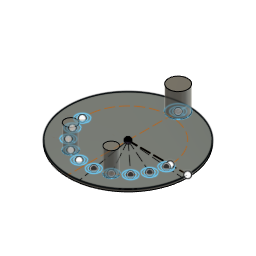
Tangible Interfaces Plate Concept (Autodesk Fusion 360 design; units mm, degrees)
Autodesk Fusion 360 part; units mm, degrees
sketch "Sketch1" plane through (0, 0, 0) normal (0, 1, 0) x (1, 0, 0)
  circle A0 centre (0, 0) radius 37.5
  line L0 (0, 37.5) -> (0, -37.5) construction
  line L1 (0, 0) -> (37.5, 0) construction
  circle A1 centre (0, 0) radius 26.5 construction
  line L2 (0, 0) -> (37.5, 0) construction
  line L3 (0, 0) -> (6.5118, -36.9303) construction
  line L4 (0, 0) -> (37.5, 0) construction
  line L5 (0, 0) -> (37.3573, -3.2683) construction
  line L6 (0, 0) -> (37.5, 0) construction
  line L7 (0, 0) -> (24.2558, -10.6728) construction
  line L8 (0, 0) -> (26.5, 0) construction
  line L9 (0, 0) -> (19.5378, -17.9031) construction
  line L10 (0, 0) -> (26.5, 0) construction
  line L11 (0, 0) -> (12.7462, -23.2333) construction
  line L12 (0, 0) -> (26.5, 0) construction
  circle A2 centre (26.3992, -2.3096) radius 2.5
  circle A3 centre (24.2558, -10.6728) radius 2.5
  circle A4 centre (19.5378, -17.9031) radius 2.5
  circle A5 centre (12.7462, -23.2333) radius 2.5
  circle A6 centre (4.6017, -26.0974) radius 2.5
  circle A7 centre (-4.6017, -26.0974) radius 2.5
  circle A8 centre (-12.7462, -23.2333) radius 2.5
  circle A9 centre (-19.5378, -17.9031) radius 2.5
  circle A10 centre (-24.2558, -10.6728) radius 2.5
  circle A11 centre (-26.3992, -2.3096) radius 2.5
  line L13 (0, 37.5) -> (0, 31.5)
  circle A12 centre (0, 31.5) radius 2.5
  circle A13 centre (-24.2558, -10.6728) radius 3.75
  circle A14 centre (24.2558, -10.6728) radius 3.75
  circle A15 centre (0, 31.5) radius 3.75
  circle A16 centre (-4.6017, -26.0974) radius 3.75
  circle A17 centre (4.6017, -26.0974) radius 3.75
  circle A18 centre (-12.7462, -23.2333) radius 3.75
  circle A19 centre (12.7462, -23.2333) radius 3.75
  circle A20 centre (-19.5378, -17.9031) radius 3.75
  circle A21 centre (-26.3992, -2.3096) radius 3.75
  circle A22 centre (26.3992, -2.3096) radius 3.75
  circle A23 centre (19.5378, -17.9031) radius 3.75
  circle A24 centre (0, 31.5) radius 6
  dimension "d1" = 75
  dimension "d5" = 80
  dimension "d6" = 5
  dimension "d9" = 23.75
  dimension "d10" = 42.5
  dimension "d11" = 61.25
  dimension "d12" = 5
  dimension "d13" = 5
  dimension "d14" = 5
  dimension "d15" = 5
  dimension "d16" = 5
  dimension "d29" = 6
  dimension "d39" = 7.5
  dimension "d40" = 7.5
  dimension "d41" = 7.5
  dimension "d44" = 7.5
  dimension "d45" = 7.5
  dimension "d46" = 7.5
  dimension "d47" = 7.5
  dimension "d52" = 7.5
  dimension "d53" = 7.5
  dimension "d58" = 7.5
  dimension "d63" = 7.5
  dimension "d66" = 12
  constraint coincident A0.centre L1.start
  constraint coincident A0 L0.start
  constraint coincident A0 L0.end
  constraint coincident A0 L1.end
  constraint perpendicular L0 L1
  constraint horizontal L2
  constraint horizontal L4
  constraint coincident A0 L3.end
  constraint horizontal L6
  constraint coincident A0 L5.end
  constraint horizontal L8
  constraint coincident A1 L7.end
  constraint horizontal L10
  constraint horizontal L12
  constraint coincident L5 A2.centre
  constraint coincident A1 A2.centre
  constraint coincident L7.end A3.centre
  constraint coincident L9.end A4.centre
  constraint coincident L11.end A5.centre
  constraint coincident A1 A6.centre
  constraint coincident L3 A6.centre
  constraint symmetric L0 A2 A11
  constraint symmetric L0 A3 A10
  constraint symmetric L0 A4 A9
  constraint symmetric L0 A5 A8
  constraint symmetric L0 A6 A7
  constraint parallel L0 L13
  constraint coincident L13.end A12.centre
  constraint concentric A10 A13
  constraint concentric A3 A14
  constraint concentric A12 A15
  constraint concentric A7 A16
  constraint concentric A6 A17
  constraint concentric A8 A18
  constraint concentric A5 A19
  constraint concentric A9 A20
  constraint concentric A11 A21
  constraint concentric A2 A22
  constraint concentric A4 A23
  constraint concentric A12 A24
  measures "d1" diameter of A0
  measures "d5" angle of L3 L4
  measures "d6" angle of L5 L6
  measures "d9" angle of L7 L8
  measures "d10" angle of L9 L10
  measures "d11" angle of L11 L12
  measures "d12" diameter of A2
  measures "d13" diameter of A3
  measures "d14" diameter of A4
  measures "d15" diameter of A5
  measures "d16" diameter of A6
  measures "d29" distance of L0.start L13.end
  measures "d39" diameter of A13
  measures "d40" diameter of A14
  measures "d41" diameter of A15
  measures "d44" diameter of A16
  measures "d45" diameter of A17
  measures "d46" diameter of A18
  measures "d47" diameter of A19
  measures "d52" diameter of A20
  measures "d53" diameter of A21
  measures "d58" diameter of A22
  measures "d63" diameter of A23
  measures "d66" diameter of A24
extrude "Extrude1" add sketch "Sketch1" against normal blind 2.5 contours A24 | A0 | A2 | A3 | A4 | A5 | A6 | A7 | A8 | A9 | A10 | A11 | A12 | A13 | A14 | A15 | A16 | A17 | A18 | A19 | A20 | A21 | A22 | A23 makes body 1
extrude "Extrude11" add sketch "Sketch1" along normal blind 15 separate body contours A12 | A15 makes body 2
extrude "Extrude16" add sketch "Sketch1" along normal blind 15 contours A24 bodies 1 2
extrude "Extrude17" cut 1 faces at (9.3028, -2.5, -10.3652) along direction (0, 1, 0) blind 1 on bodies 1 bodies 1
extrude "Extrude21" add sketch "Sketch1" along normal blind 15 contours A5 | A8 | A18 | A19 bodies 1
sketch "Sketch4" plane through (0, 0, 0) normal (0, 0, 1) x (1, 0, 0)
